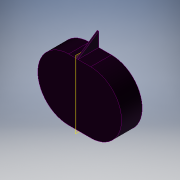
# Autodesk Inventor part: EspritOvalPool
Saved by Autodesk Inventor 2019 (Build 230136000, 136)
## iProperties
Created: 2021-06-08
Part Number: EspritOvalPool
Material: Generic
Document SubType Name: Modeling
Designer: jamieson-bl
Density: 1 g/cm^3
Appearance: Default
Author: jamieson-bl
Autodesk Inventor part; units mm, degrees
ref_plane "XZ Plane" through (0, 0, 0) normal (0, 1, 0) x (-1, 0, 0)
ref_plane "XY Plane" through (0, 0, 0) normal (0, 0, 1) x (1, 0, 0)
sketch "Sketch4" plane through (0, 0, 0) normal (0, 0, 1) x (1, 0, 0)
  arc A0 (0, 1981.2) -> (0, -1981.2) centre (0, 0) ccw
  arc A1 (1422.4, -1981.2) -> (1422.4, 1981.2) centre (1422.4, 0) ccw
  line L0 (0, 1981.2) -> (1422.4, 1981.2)
  line L1 (0, -1981.2) -> (1603.6466, -1981.2)
  dimension "d12" = 3962.4
  dimension "d13" = 3962.4
  constraints: 4 end point, 4 point on circle, 2 centre point, 1 coincident, 1 horizontal, 1 point on line, 1 tangent
  measures "d12" diameter of A0
  measures "d13" diameter of A1
extrude "Extrusion3" add sketch "Sketch4" along normal blind 12.7
sketch "Sketch6" plane through (0, 0, 12.7) normal (0, 0, 1) x (1, 0, 0)
  arc A0 (0, 1981.2) -> (0, -1981.2) centre (0, 0) ccw projected
  arc A1 (0, 1981.2) -> (0, -1981.2) centre (0, 0) ccw
  line L0 (0, -1981.2) -> (1422.4, -1981.2) projected
  arc A2 (1422.4, -1981.2) -> (1422.4, 1981.2) centre (1422.4, 0) ccw projected
  arc A3 (1422.4, -1981.2) -> (1422.4, 1981.2) centre (1422.4, 0) ccw
  line L1 (0, 1981.2) -> (1422.4, 1981.2)
  line L2 (0, -1981.2) -> (1422.4, -1981.2)
  arc A4 (0, 1968.5) -> (0, -1968.5) centre (0, 0) ccw
  arc A5 (1422.4, -1968.5) -> (1422.4, 1968.5) centre (1422.4, 0) ccw
  line L3 (1422.4, 0) -> (1422.4, -1968.5) construction
  line L4 (1422.4, 0) -> (3390.9, 0) construction
  line L5 (0, 1968.5) -> (1422.4, 1968.5)
  line L6 (0, -1968.5) -> (1422.4, -1968.5)
  dimension "d18" = 1968.5
  dimension "d19" = 1968.5
  dimension "d20" = 90
  constraints: 12 end point, 11 point on circle, 4 centre point, 4 horizontal, 3 coincident, 1 parallel, 1 perpendicular
  measures "d18" radius of A4
  measures "d19" radius of A5
  measures "d20" angle of L3 L4
extrude "Extrusion4" add sketch "Sketch6" along normal blind 1320.8 contours L1 A2 L0 A0 | L5 A5 L6 A4
ref_plane "Work Plane1" through (508, 0, 0) normal (1, 0, 0) x (0, 1, 0)
sketch "Sketch8" plane through (508, 0, 0) normal (1, 0, 0) x (0, 1, 0)
  line L0 (1981.2, 0) -> (1981.2, 1333.5) projected
  line L1 (1981.2, 0) -> (2895.6, 0)
  line L2 (2895.6, 0) -> (1981.2, 1333.5)
  line L3 (1981.2, 1333.5) -> (1981.2, 0)
  line L4 (1981.2, 1333.5) -> (1981.2, 0)
  point P0 (0, 0)
  dimension "d24" = 914.4
  constraints: 8 end point, 2 collinear, 1 horizontal
  measures "d24" distance of L0.start L1.end
extrude "Extrusion5" add sketch "Sketch8" along normal blind 101.6
mirror "Mirror1" about plane through (0, 0, 0) normal (0, 1, 0) of "Extrusion5"
body "Solid2"
